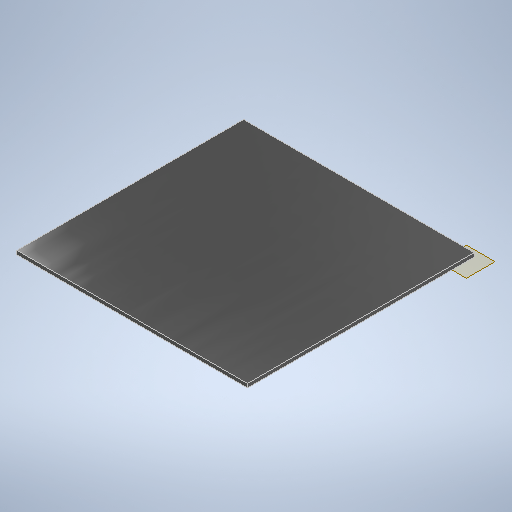
# Autodesk Inventor part: Lid
Saved by Autodesk Inventor 2025 (Build 290162000, 162)
## iProperties
Created: 2024-08-10
Part Number: Lid
Material: Generic
Document SubType Name: Modeling
Designer: ethan
Density: 1 g/cm^3
Appearance: Dark Gray
Author: ethan
Autodesk Inventor part; units mm, degrees
ref_plane "YZ Plane" through (0, 0, 0) normal (1, 0, 0) x (0, 1, 0)
ref_plane "XZ Plane" through (0, 0, 0) normal (0, 1, 0) x (-1, 0, 0)
ref_plane "XY Plane" through (0, 0, 0) normal (0, 0, 1) x (1, 0, 0)
ref_plane "Work Plane1" through (0, 86, 164.5) normal (0, 1, 0) x (1, 0, 0)
sketch "Sketch7" plane through (0, 86, 164.5) normal (0, 1, 0) x (1, 0, 0)
  line L0 (-3, 170.5) -> (5, 170.5) construction
  line L1 (-3, 170.5) -> (-3, -3) construction
  line L2 (173.5, -3) -> (-3, -3) construction
  line L3 (173.5, 170.5) -> (173.5, -3) construction
  line L4 (165.5, 170.5) -> (173.5, 170.5) construction
  line L5 (165.5, 170.5) -> (165.5, 167.3) construction
  line L6 (170.5, 167.3) -> (165.5, 167.3) construction
  line L7 (170.5, 167.3) -> (170.5, 164.5) construction
  line L8 (170.5, 164.5) -> (165.5, 164.5) construction
  line L9 (165.5, 164.5) -> (165.5, 160.5) construction
  line L10 (170.5, 160.5) -> (165.5, 160.5) construction
  line L11 (170.5, 160.5) -> (170.5, 0) construction
  line L12 (170.5, 0) -> (0, 0) construction
  line L13 (0, 0) -> (0, 160.5) construction
  line L14 (5, 160.5) -> (0, 160.5) construction
  line L15 (5, 164.5) -> (5, 160.5) construction
  line L16 (5, 164.5) -> (0, 164.5) construction
  line L17 (0, 164.5) -> (0, 167.3) construction
  line L18 (5, 167.3) -> (0, 167.3) construction
  line L19 (5, 170.5) -> (5, 167.3) construction
  line L20 (165.3, 160.3) -> (165.3, 164.7) construction
  line L21 (165.3, 164.7) -> (170.3, 164.7) construction
  line L22 (170.3, 164.7) -> (170.3, 167.1) construction
  line L23 (170.3, 167.1) -> (165.3, 167.1) construction
  line L24 (165.3, 167.1) -> (165.3, 170.7) construction
  line L25 (165.3, 170.7) -> (173.7, 170.7) construction
  line L26 (173.7, 170.7) -> (173.7, -3.2) construction
  line L27 (173.7, -3.2) -> (-3.2, -3.2) construction
  line L28 (-3.2, -3.2) -> (-3.2, 170.7) construction
  line L29 (-3.2, 170.7) -> (5.2, 170.7) construction
  line L30 (5.2, 170.7) -> (5.2, 167.1) construction
  line L31 (5.2, 167.1) -> (0.2, 167.1) construction
  line L32 (0.2, 167.1) -> (0.2, 164.7) construction
  line L33 (0.2, 164.7) -> (5.2, 164.7) construction
  line L34 (5.2, 164.7) -> (5.2, 160.3) construction
  line L35 (5.2, 160.3) -> (0.2, 160.3) construction
  line L36 (0.2, 160.3) -> (0.2, 0.2) construction
  line L37 (0.2, 0.2) -> (170.3, 0.2) construction
  line L38 (170.3, 0.2) -> (170.3, 160.3) construction
  line L39 (170.3, 160.3) -> (165.3, 160.3) construction
  line L40 (170.3, 160.3) -> (0.2, 160.3)
  line L41 (0.2, 160.3) -> (0.2, 0.2)
  line L42 (0.2, 0.2) -> (170.3, 0.2)
  line L43 (170.3, 0.2) -> (170.3, 160.3)
  point P0 (0, 164.5)
  dimension "d18" = 0.2
  constraints: 48 end point, 2 parallel, 1 horizontal, 1 perpendicular, 19 other
  measures "d18" distance between parallel lines of L10 L39
extrude "Extrusion7" add sketch "Sketch7" along normal blind 3
sketch "Sketch8" plane through (0, 89, 164.5) normal (0, 1, 0) x (1, 0, 0)
  line L0 (-3, 170.5) -> (5, 170.5) construction
  line L1 (-3, 170.5) -> (-3, -3) construction
  line L2 (173.5, -3) -> (-3, -3) construction
  line L3 (173.5, 170.5) -> (173.5, -3) construction
  line L4 (165.5, 170.5) -> (173.5, 170.5) construction
  line L5 (165.5, 170.5) -> (165.5, 167.3) construction
  line L6 (170.5, 167.3) -> (165.5, 167.3) construction
  line L7 (170.5, 167.3) -> (170.5, 164.5) construction
  line L8 (170.5, 164.5) -> (165.5, 164.5) construction
  line L9 (165.5, 164.5) -> (165.5, 160.5) construction
  line L10 (170.5, 160.5) -> (165.5, 160.5) construction
  line L11 (170.5, 160.5) -> (170.5, 0) construction
  line L12 (170.5, 0) -> (0, 0) construction
  line L13 (0, 0) -> (0, 160.5) construction
  line L14 (5, 160.5) -> (0, 160.5) construction
  line L15 (5, 164.5) -> (5, 160.5) construction
  line L16 (5, 164.5) -> (0, 164.5) construction
  line L17 (0, 164.5) -> (0, 167.3) construction
  line L18 (5, 167.3) -> (0, 167.3) construction
  line L19 (5, 170.5) -> (5, 167.3) construction
  line L20 (173.5, 170.5) -> (-3, 170.5) construction
  line L21 (-3, 170.5) -> (-3, -3) construction
  line L22 (-3, -3) -> (173.5, -3) construction
  line L23 (173.5, -3) -> (173.5, 170.5) construction
  line L24 (173.5, 170.5) -> (-3, 170.5)
  line L25 (-3, 170.5) -> (-3, -3)
  line L26 (-3, -3) -> (173.5, -3)
  line L27 (173.5, -3) -> (173.5, 170.5)
  point P0 (0, 164.5)
  constraints: 16 end point, 4 parallel, 2 horizontal, 2 perpendicular
extrude "Extrusion8" add sketch "Sketch8" along normal blind 3
body "Solid1"
